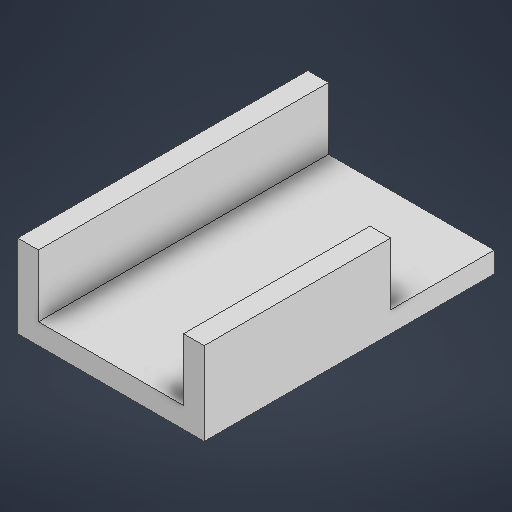
# Autodesk Inventor part: outlifting
Saved by Autodesk Inventor 2026.2 (Build 302298000, 298)
## iProperties
Created: 2026-04-16
Part Number: outlifting
Material: Generic
Document SubType Name: Modeling
Designer: danda
Density: 1 g/cm^3
Appearance: Default
Author: danda
Autodesk Inventor part; units mm, degrees
ref_plane "YZ Plane" through (0, 0, 0) normal (1, 0, 0) x (0, 1, 0)
ref_plane "XZ Plane" through (0, 0, 0) normal (0, 1, 0) x (-1, 0, 0)
ref_plane "XY Plane" through (0, 0, 0) normal (0, 0, 1) x (1, 0, 0)
sketch "Sketch1" plane through (0, 0, 0) normal (0, 0, 1) x (1, 0, 0)
  line L0 (14.4828, 12.3536) -> (49.4828, 12.3536)
  line L1 (49.4828, 12.3536) -> (49.4828, 27.3536)
  line L2 (14.4828, 12.3536) -> (14.4828, 27.3536)
  line L3 (54.4828, 27.3536) -> (54.4828, 7.3536)
  line L4 (54.4828, 7.3536) -> (9.4828, 7.3536)
  line L5 (9.4828, 7.3536) -> (9.4828, 27.3536)
  line L6 (9.4828, 27.3536) -> (14.4828, 27.3536)
  line L7 (49.4828, 27.3536) -> (54.4828, 27.3536)
  point P0 (0, 0)
  dimension "d0" = 35
  dimension "d1" = 15
  dimension "d2" = 15
  dimension "d3" = 5
  constraints: 16 end point, 2 horizontal, 2 perpendicular, 1 collinear, 1 vertical, 2 other
  measures "d0" distance of L0.start L0.end
  measures "d1" distance of L0.end L1.end
  measures "d2" distance of L0.start L2.end
  measures "d3" distance between parallel lines of L0 L4
extrude "Extrusion1" add sketch "Sketch1" along normal blind 70
sketch "Sketch3" plane through (54.4828, 7.3536, 0) normal (1, 0, 0) x (0, 0, -1)
  line L0 (0, 20) -> (0, 0) projected
  line L1 (0, 5) -> (-70, 5) projected
  line L2 (0, 20) -> (-25, 20)
  line L3 (-25, 20) -> (-25, 5)
  line L4 (-25, 5) -> (0, 5)
  line L5 (0, 5) -> (0, 20)
  point P0 (0, -7.3536)
  dimension "d6" = 25
  constraints: 8 end point, 2 parallel, 1 horizontal, 1 perpendicular, 1 point on line
  measures "d6" distance of L4.end L3.end
extrude "Extrusion2" cut sketch "Sketch3" against normal blind 5
body "Solid1"
